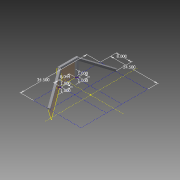
# Autodesk Inventor part: Roll Bar
Saved by Autodesk Inventor 2015 (Build 190159000, 159)
## iProperties
Created: 2016-01-20
Part Number: Roll Bar
Material: Generic
Document SubType Name: Modeling
Designer: sethbattis
Density: 1 g/cm^3
Appearance: Default
Author: sethbattis
Autodesk Inventor part; units mm, degrees
ref_plane "YZ Plane" through (0, 0, 0) normal (1, 0, 0) x (0, 1, 0)
ref_plane "XZ Plane" through (0, 0, 0) normal (0, 1, 0) x (-1, 0, 0)
ref_plane "XY Plane" through (0, 0, 0) normal (0, 0, 1) x (1, 0, 0)
sketch "Sketch3" plane through (0, 0, 0) normal (0, 1, 0) x (-1, 0, 0)
  line L0 (311.15, 438.15) -> (-311.15, 438.15) construction
  line L1 (-311.15, 438.15) -> (-311.15, -438.15) construction
  line L2 (-311.15, -438.15) -> (311.15, -438.15) construction
  line L3 (311.15, -438.15) -> (311.15, 438.15) construction
  line L4 (0, -613.41) -> (0, 613.41) construction
  line L5 (435.61, 0) -> (-435.61, 0) construction
  line L6 (107.95, 438.15) -> (107.95, -438.15) construction
  line L7 (311.15, 102.1588) -> (-311.15, 102.1588) construction
  line L8 (311.15, -102.1588) -> (-311.15, -102.1588) construction
  line L9 (311.15, 127.5588) -> (285.75, 127.5588)
  line L10 (285.75, 127.5588) -> (285.75, 102.1588)
  line L11 (285.75, 102.1588) -> (311.15, 102.1588)
  line L12 (311.15, 102.1588) -> (311.15, 127.5588)
  line L13 (311.15, -102.1588) -> (285.75, -102.1588)
  line L14 (285.75, -102.1588) -> (285.75, -127.5588)
  line L15 (285.75, -127.5588) -> (311.15, -127.5588)
  line L16 (311.15, -127.5588) -> (311.15, -102.1588)
  point P0 (0, 0)
  dimension "d8" = 876.3
  dimension "d9" = 622.3
  dimension "d10" = 203.2
  dimension "d11" = 204.3176
  dimension "d12" = 25.4
  dimension "d13" = 25.4
  dimension "d14" = 25.4
  dimension "d15" = 25.4
  constraints: 30 end point, 7 point on line, 6 parallel, 4 horizontal, 4 perpendicular, 3 collinear, 1 vertical, 3 other
  measures "d8" distance of L2.end L0.start
  measures "d9" distance of L1.end L2.end
  measures "d10" distance between parallel lines of L3 L6
  measures "d11" distance between parallel lines of L8 L7
  measures "d12" distance of L11.end L10.end
  measures "d13" distance of L10.end L9.end
  measures "d14" distance of L15.end L14.end
  measures "d15" distance of L14.end L13.end
extrude "Extrusion1" add sketch "Sketch3" along normal blind 203.2
ref_plane "Work Plane1" through (-285.75, 203.2, 127.5588) normal (0.8678585, 0, -0.4968114) x (0.4320296, -0.4937482, 0.7546941)
sketch "Sketch4" plane through (-285.75, 203.2, 127.5588) normal (0.8678585, 0, -0.4968114) x (0.4320296, -0.4937482, 0.7546941)
  line L0 (-19.8109, -14.5079) -> (410.9042, -25.3919)
  line L1 (410.9042, -25.3919) -> (411.5458, 0)
  line L2 (411.5458, 0) -> (-19.1692, 10.884)
  line L3 (-19.1692, 10.884) -> (-19.8109, -14.5079)
  line L4 (323.7574, 49.8449) -> (592.6095, -102.8051) construction
  line L5 (411.5458, 0) -> (-249.7926, 375.4977) construction
  point P0 (127.5142, 161.2687)
  dimension "d18" = 25.4
  constraints: 8 end point, 2 parallel, 1 coincident, 1 perpendicular
  measures "d18" distance of L1.end L0.end
extrude "Extrusion2" add sketch "Sketch4" along normal mid plane 25.4
mirror "Mirror1" about plane through (0, 0, 0) normal (0, 0, 1) of "Extrusion2"
ref_plane "Work Plane2" through (-311.15, 203.2, -127.5588) normal (1, 0, 0) x (0, 0, 1)
sketch "Sketch5" plane through (-311.15, 203.2, -127.5588) normal (1, 0, 0) x (0, 0, 1)
  line L0 (0, 0) -> (255.1176, 0)
  line L1 (255.1176, 0) -> (255.1176, -25.4)
  line L2 (255.1176, -25.4) -> (0, -25.4)
  line L3 (0, -25.4) -> (0, 0)
  point P0 (127.5588, 203.2)
  dimension "d21" = 25.4
  constraints: 8 end point, 2 parallel, 1 coincident, 1 horizontal, 1 perpendicular
  measures "d21" distance of L0.end L1.end
extrude "Extrusion3" add sketch "Sketch5" along normal blind 25.4
body "Solid2"
